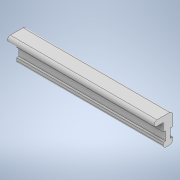
# Autodesk Inventor part: Rails
Saved by Autodesk Inventor 2020 (Build 240168000, 168)
## iProperties
Created: 2020-07-03
Part Number: Rails
Material: Generic
Document SubType Name: Modeling
Designer: lukep
Density: 1 g/cm^3
Appearance: Default
Author: lukep
Autodesk Inventor part; units mm, degrees
ref_plane "YZ Plane" through (0, 0, 0) normal (1, 0, 0) x (0, 1, 0)
ref_plane "XZ Plane" through (0, 0, 0) normal (0, 1, 0) x (-1, 0, 0)
ref_plane "XY Plane" through (0, 0, 0) normal (0, 0, 1) x (1, 0, 0)
sketch "Sketch1" plane through (0, 0, 0) normal (0, 1, 0) x (-1, 0, 0)
  line L0 (0, 0) -> (80, 0)
  line L1 (80, 0) -> (80, -5)
  line L2 (80, -5) -> (0, -5)
  line L3 (0, -5) -> (0, 0)
  dimension "d0" = 5
  dimension "d1" = 80
  constraints: 8 end point, 2 parallel, 1 horizontal, 1 perpendicular
  measures "d0" distance of L0.end L1.end
  measures "d1" distance of L1.end L2.end
extrude "Extrusion1" add sketch "Sketch1" along normal blind 3
sketch "Sketch2" plane through (0, 3, 0) normal (0, 1, 0) x (1, 0, 0)
  line L0 (0, 3.825) -> (-80, 3.825)
  line L1 (-80, 3.825) -> (-80, 1.175)
  line L2 (-80, 1.175) -> (0, 1.175)
  line L3 (0, 1.175) -> (0, 3.825)
  line L4 (0, 3.825) -> (-80, 1.175) construction
  line L5 (-80, 3.825) -> (0, 1.175) construction
  line L6 (0, 0) -> (0, 5) projected
  line L7 (-80, 5) -> (-80, 0) projected
  point P0 (-40, 2.5)
  point P1 (0, 2.5)
  point P2 (0, 2.5)
  dimension "d4" = 2.65
  constraints: 12 end point, 4 midpoint, 2 collinear, 2 parallel, 1 coincident, 1 horizontal, 1 perpendicular
  measures "d4" distance of L2.end L0.start
extrude "Extrusion2" add sketch "Sketch2" along normal blind 4.826
sketch "Sketch3" plane through (0, 0, 0) normal (1, 0, 0) x (0, 0, -1)
  line L0 (5, 7.826) -> (0, 7.826)
  line L1 (0, 7.826) -> (0, 15.326)
  line L2 (0, 15.326) -> (5, 15.326)
  line L3 (5, 15.326) -> (5, 7.826)
  line L4 (1.175, 7.826) -> (3.825, 7.826) projected
  line L5 (5, 0) -> (5, 3) projected
  line L6 (0, 0) -> (0, 3) projected
  line L7 (0, 15.326) -> (-5, 15.326)
  line L8 (-5, 15.326) -> (-5, 12.326)
  line L9 (-5, 12.326) -> (0, 12.326)
  line L10 (0, 12.326) -> (0, 15.326)
  dimension "d7" = 7.5
  dimension "d8" = 3
  dimension "d9" = 5
  constraints: 16 end point, 4 parallel, 3 collinear, 2 horizontal, 2 perpendicular
  measures "d7" distance of L2.end L0.start
  measures "d8" distance of L7.end L8.end
  measures "d9" distance of L8.end L9.end
extrude "Extrusion3" add sketch "Sketch3" against normal up to surface (80 mm away)
fillet "Fillet1" radius 1.5 3 edges at (-40, 15.326, -5) (-40, 15.326, 5) (-40, 12.326, 5)
fillet "Fillet2" radius 1.5 2 edges at (-40, 0, 0) (-40, 0, -5)
body "Solid1"
